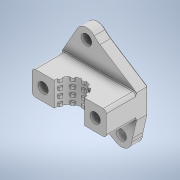
# Autodesk Inventor part: Extruder-Motherboard Cable Harness
Saved by Autodesk Inventor 2020 (Build 240168000, 168)
## iProperties
Created: 2019-12-22
Part Number: Extruder-Motherboard Cable Harness
Material: Generic
Document SubType Name: Modeling
Designer: pepd9
Density: 1 g/cm^3
Appearance: Default
Author: pepd9
Autodesk Inventor part; units mm, degrees
ref_plane "YZ Plane" through (0, 0, 0) normal (1, 0, 0) x (0, 1, 0)
ref_plane "XZ Plane" through (0, 0, 0) normal (0, 1, 0) x (-1, 0, 0)
ref_plane "XY Plane" through (0, 0, 0) normal (0, 0, 1) x (1, 0, 0)
ref_plane "Work Plane1" through (0, 0, 0) normal (0, 0, 1) x (1, 0, 0)
sketch "Sketch1" plane through (0, 0, 0) normal (0, 0, 1) x (1, 0, 0)
  circle A0 centre (228, 110.5) radius 1.1 construction
  circle A1 centre (239.5, 89) radius 1.1 construction
  line L0 (220, 118.5) -> (244.5, 118.5)
  line L1 (244.5, 118.5) -> (244.5, 81)
  line L2 (244.5, 81) -> (220, 81)
  line L3 (220, 81) -> (220, 118.5)
  point P0 (0, 0)
  dimension "d0" = 5
  dimension "d1" = 8
  dimension "d2" = 8
  dimension "d3" = 8
  constraints: 8 end point, 2 parallel, 1 horizontal, 1 perpendicular
  measures "d0" distance from line of A1.centre L1
  measures "d1" distance from line of L3 A0.centre
  measures "d2" distance from line of L2 A1.centre
  measures "d3" distance from line of L0 A0.centre
extrude "Extrusion1" add sketch "Sketch1" along normal blind 3
sketch "Sketch2" plane through (0, 0, 3) normal (0, 0, 1) x (1, 0, 0)
  circle A0 centre (228, 110.5) radius 1.1 projected
  circle A1 centre (239.5, 89) radius 1.1 projected
  point P0 (0, 0)
hole "Hole1" at (228, 110.5, 3) at (239.5, 89, 3) direction (0, 0, -1) diameter 3.4 end through all clearance for "Socket Head Cap Screw" size "M3" standard "Ansi Metric M Profile"
ref_plane "Work Plane2" through (220, 103.5, 0) normal (0, 1, 0) x (1, 0, 0)
sketch "Sketch3" plane through (220, 103.5, 0) normal (0, 1, 0) x (1, 0, 0)
  line L0 (0, -3) -> (24.5, -3) projected
  line L1 (12.25, -3) -> (12.25, -35.3077) construction
  circle A0 centre (12.25, -13) radius 5
  line L2 (24.5, -13) -> (24.5, -3)
  line L3 (7.25, -13) -> (0, -13)
  line L4 (0, -13) -> (0, -3)
  line L5 (0, -13) -> (24.5, -13)
  point P0 (-220, 0)
  point P1 (17.25, -13)
  dimension "d14" = 10
  dimension "d15" = 10
  dimension "d18" = 10
  constraints: 10 end point, 3 vertical, 2 horizontal, 1 horizontal alignment, 1 midpoint, 1 point on line, 3 other
  measures "d15" distance from line of L0 point (12.25, -13)
  measures "d18" distance of L3.end L0.start
extrude "Extrusion2" add sketch "Sketch3" against normal blind 8 contours L0 L2 L5 A0 L3 L4
sketch "Sketch4" plane through (237.25, 103.5, 13) normal (0, 0, 1) x (1, 0, 0)
  line L0 (-17.25, 0) -> (-10, 0) projected
  line L1 (-17.25, 0) -> (-17.25, -8) projected
  line L2 (-10, -8) -> (-17.25, -8) projected
  line L3 (-10, 0) -> (-10, -8) projected
  line L4 (0, 0) -> (7.25, 0) projected
  line L5 (0, 0) -> (0, -8) projected
  line L6 (7.25, -8) -> (0, -8) projected
  line L7 (7.25, 0) -> (7.25, -8) projected
  point P0 (-237.25, -103.5)
  point P1 (-13.625, -4)
  point P2 (3.625, -4)
hole "Hole2" at (223.625, 99.5, 13) at (240.875, 99.5, 13) direction (0, 0, -1) diameter 3.4 end through all clearance for "Socket Head Cap Screw" size "M3" standard "Ansi Metric M Profile"
sketch "Sketch5" plane through (0, 0, 0) normal (0, 0, -1) x (-1, 0, 0)
  circle A0 centre (-240.875, 99.5) radius 1.7 projected
  circle A1 centre (-223.625, 99.5) radius 1.7 projected
  line L0 (-243.625, 101.0877) -> (-240.875, 102.6754)
  line L1 (-240.875, 102.6754) -> (-238.125, 101.0877)
  line L2 (-238.125, 101.0877) -> (-238.125, 97.9123)
  line L3 (-238.125, 97.9123) -> (-240.875, 96.3246)
  line L4 (-240.875, 96.3246) -> (-243.625, 97.9123)
  line L5 (-243.625, 97.9123) -> (-243.625, 101.0877)
  line L6 (-226.375, 101.0877) -> (-223.625, 102.6754)
  line L7 (-223.625, 102.6754) -> (-220.875, 101.0877)
  line L8 (-220.875, 101.0877) -> (-220.875, 97.9123)
  line L9 (-220.875, 97.9123) -> (-223.625, 96.3246)
  line L10 (-223.625, 96.3246) -> (-226.375, 97.9123)
  line L11 (-226.375, 97.9123) -> (-226.375, 101.0877)
  point P0 (0, 0)
  point P1 (-223.625, 99.5)
  dimension "d28" = 5.5
  dimension "d29" = 5.5
  constraints: 24 end point, 2 coincident, 26 other
  measures "d28" distance between parallel lines of L5 L2
  measures "d29" distance between parallel lines of L8 L11
extrude "Extrusion3" cut sketch "Sketch5" against normal blind 5
sketch "Sketch6" plane through (220, 103.5, 0) normal (0, 1, 0) x (1, 0, 0)
  line L0 (0, -3) -> (0, -13) projected
  line L1 (0, -13) -> (7.25, -13) projected
  arc A0 (17.25, -13) -> (7.25, -13) centre (12.25, -13) ccw projected
  line L2 (17.25, -13) -> (24.5, -13) projected
  line L3 (24.5, -13) -> (24.5, -3) projected
  line L4 (0, -3) -> (24.5, -3) projected
  line L5 (7.348, -12.015) -> (7.8461, -11.9714)
  line L6 (7.8461, -11.9714) -> (8.1881, -11.0317)
  line L7 (8.1881, -11.0317) -> (7.8051, -10.7103)
  point P0 (-220, 0)
  dimension "d32" = 5
  dimension "d33" = 45
  dimension "d34" = 115
  dimension "d35" = 1
  dimension "d36" = 0.5
  dimension "d37" = 0.5
  constraints: 6 end point, 2 point on circle
  measures "d32" angle of L5 L1
  measures "d33" angle of L5 L7
  measures "d34" angle of L6 L5
  measures "d35" distance of L5.end L6.end
  measures "d36" distance of L5.start L5.end
  measures "d37" distance of L6.end L7.end
extrude "Extrusion4" add sketch "Sketch6" against normal blind 1 contours A0 L7 L6 L5
pattern_circular "Circular Pattern1" count 5 over 140 about axis through (232.25, 103.5, 13) along (0, -1, 0) of "Extrusion4"
pattern_linear "Rectangular Pattern1" count 4 spacing 2.3 along (0, -1, 0) of "Extrusion4", "Circular Pattern1"
sketch "Sketch7" plane through (0, 0, 3) normal (0, 0, 1) x (1, 0, 0)
  line L0 (220, 103.5) -> (244.5, 103.5) projected
  line L1 (244.5, 103.5) -> (244.5, 118.5) projected
  line L2 (244.5, 118.5) -> (220, 118.5) projected
  line L3 (220, 118.5) -> (220, 103.5) projected
  circle A0 centre (228, 110.5) radius 1.7 projected
  circle A1 centre (239.5, 89) radius 1.7 projected
  line L4 (244.5, 95.5) -> (220, 95.5) projected
  line L5 (220, 95.5) -> (220, 81) projected
  line L6 (220, 81) -> (244.5, 81) projected
  line L7 (244.5, 81) -> (244.5, 95.5) projected
  circle A2 centre (228, 110.5) radius 1.7 projected
  circle A3 centre (228, 110.5) radius 3.5
  circle A4 centre (239.5, 89) radius 3.5
  line L8 (220, 118.5) -> (220, 103.5) projected
  line L9 (244.5, 103.5) -> (231.0594, 112.2)
  line L10 (224.9565, 112.2283) -> (220, 103.5)
  line L11 (244.5, 95.5) -> (220, 95.5) projected
  line L12 (220, 95.5) -> (237.844, 85.9166)
  line L13 (243, 89) -> (244.5, 95.5)
  point P0 (0, 0)
  dimension "d46" = 7
  dimension "d47" = 7
  constraints: 8 end point, 4 point on circle, 2 centre point, 2 coincident, 2 tangent
  measures "d46" diameter of A3
  measures "d47" diameter of A4
extrude "Extrusion5" cut sketch "Sketch7" against normal through all contours L3 L2 L1 L9 A3 L10 | L7 L6 L5 L12 A4 L13
fillet "Fillet1" radius 10 2 edges at (231.0594, 112.2, 1.5) (243, 89, 1.5)
fillet "Fillet2" radius 1 4 edges at (244.5, 103.5, 8) (244.5, 95.5, 8) (220, 95.5, 8) (220, 103.5, 8)
sketch "Sketch8" plane through (0, 0, 5) normal (0, 0, -1) x (-1, 0, 0)
  line L0 (-240.875, 96.3246) -> (-243.625, 97.9123) projected
  line L1 (-238.125, 97.9123) -> (-240.875, 96.3246) projected
  line L2 (-238.125, 101.0877) -> (-238.125, 97.9123) projected
  line L3 (-240.875, 102.6754) -> (-238.125, 101.0877) projected
  line L4 (-243.625, 101.0877) -> (-240.875, 102.6754) projected
  line L5 (-243.625, 97.9123) -> (-243.625, 101.0877) projected
  circle A0 centre (-240.875, 99.5) radius 1.7 projected
  line L6 (-220.875, 97.9123) -> (-223.625, 96.3246) projected
  line L7 (-220.875, 101.0877) -> (-220.875, 97.9123) projected
  line L8 (-223.625, 102.6754) -> (-220.875, 101.0877) projected
  line L9 (-226.375, 101.0877) -> (-223.625, 102.6754) projected
  line L10 (-226.375, 97.9123) -> (-226.375, 101.0877) projected
  line L11 (-223.625, 96.3246) -> (-226.375, 97.9123) projected
  circle A1 centre (-223.625, 99.5) radius 1.7 projected
  line L12 (-235.6121, 101.2) -> (-234.4702, 101.2) projected
  line L13 (-246.7088, 97.8) -> (-235.0412, 97.8)
  line L14 (-235.0412, 97.8) -> (-235.0412, 101.2)
  line L15 (-235.0412, 101.2) -> (-246.7088, 101.2)
  line L16 (-246.7088, 101.2) -> (-246.7088, 97.8)
  line L17 (-246.7088, 97.8) -> (-235.0412, 101.2) construction
  line L18 (-235.0412, 97.8) -> (-246.7088, 101.2) construction
  line L19 (-219.1294, 97.8) -> (-228.1206, 97.8)
  line L20 (-228.1206, 97.8) -> (-228.1206, 101.2)
  line L21 (-228.1206, 101.2) -> (-219.1294, 101.2)
  line L22 (-219.1294, 101.2) -> (-219.1294, 97.8)
  line L23 (-219.1294, 97.8) -> (-228.1206, 101.2) construction
  line L24 (-228.1206, 97.8) -> (-219.1294, 101.2) construction
  line L25 (-237.844, 85.9166) -> (-220, 95.5) projected
  line L26 (-220, 103.5) -> (-220, 95.5) projected
  line L27 (-220, 103.5) -> (-224.9565, 112.2283) projected
  arc A2 (-224.9565, 112.2283) -> (-230.563, 112.8835) centre (-228, 110.5) ccw projected
  arc A3 (-232.4521, 111.2985) -> (-230.563, 112.8835) centre (-237.886, 119.6933) ccw projected
  line L28 (-232.4521, 111.2985) -> (-244.5, 103.5) projected
  line L29 (-244.5, 95.5) -> (-244.5, 103.5) projected
  line L30 (-244.5, 95.5) -> (-243.1723, 89.7464) projected
  arc A4 (-242.9783, 88.6106) -> (-243.1723, 89.7464) centre (-252.9162, 87.4978) ccw projected
  arc A5 (-242.9783, 88.6106) -> (-237.844, 85.9166) centre (-239.5, 89) ccw projected
  line L31 (-220.875, 101.0877) -> (-220.875, 97.9123) projected
  line L32 (-220.875, 97.9123) -> (-223.625, 96.3246) projected
  line L33 (-223.625, 96.3246) -> (-226.375, 97.9123) projected
  line L34 (-226.375, 97.9123) -> (-226.375, 101.0877) projected
  line L35 (-226.375, 101.0877) -> (-223.625, 102.6754) projected
  line L36 (-223.625, 102.6754) -> (-220.875, 101.0877) projected
  line L37 (-238.125, 97.9123) -> (-240.875, 96.3246) projected
  line L38 (-240.875, 96.3246) -> (-243.625, 97.9123) projected
  line L39 (-243.625, 97.9123) -> (-243.625, 101.0877) projected
  line L40 (-243.625, 101.0877) -> (-240.875, 102.6754) projected
  line L41 (-240.875, 102.6754) -> (-238.125, 101.0877) projected
  line L42 (-238.125, 101.0877) -> (-238.125, 97.9123) projected
  circle A6 centre (-228, 110.5) radius 1.7 projected
  circle A7 centre (-239.5, 89) radius 1.7 projected
  point P0 (0, 0)
  point P1 (-223.625, 99.5)
  point P2 (-223.625, 101.2)
  point P3 (-226.1805, 101.2)
  point P4 (-226.1805, 97.8)
  point P5 (-223.625, 97.8)
  point P6 (-221.0695, 101.2)
  point P7 (-221.0695, 97.8)
  point P8 (-238.3195, 101.2)
  point P9 (-240.875, 101.2)
  point P10 (-240.875, 97.8)
  point P11 (-238.3195, 97.8)
  point P12 (-243.4305, 101.2)
  point P13 (-243.4305, 97.8)
  dimension "d52" = 3.4
  dimension "d53" = 3.4
  constraints: 24 end point, 5 midpoint, 4 parallel, 2 horizontal, 2 perpendicular
  measures "d52" distance of L14.end L13.end
  measures "d53" distance of L19.end L20.end
extrude "Extrusion6" cut sketch "Sketch8" against normal blind 0.5 contours L0 L5 L4 L15 A0 L13 | L13 A0 L15 L3 L2 L1 | L19 A1 L21 L8 L7 L6 | L19 L11 L10 L9 L21 A1
sketch "Sketch9" plane through (0, 0, 5.5) normal (0, 0, -1) x (-1, 0, 0)
  line L0 (-240.875, 101.2) -> (-238.3195, 101.2) projected
  arc A0 (-240.875, 97.8) -> (-240.875, 101.2) centre (-240.875, 99.5) ccw projected
  line L1 (-238.3195, 97.8) -> (-240.875, 97.8) projected
  line L2 (-238.125, 97.9123) -> (-238.3195, 97.8) projected
  line L3 (-238.125, 101.0877) -> (-238.125, 97.9123) projected
  line L4 (-238.3195, 101.2) -> (-238.125, 101.0877) projected
  line L5 (-243.4305, 101.2) -> (-240.875, 101.2) projected
  line L6 (-243.625, 101.0877) -> (-243.4305, 101.2) projected
  line L7 (-243.625, 97.9123) -> (-243.625, 101.0877) projected
  line L8 (-243.4305, 97.8) -> (-243.625, 97.9123) projected
  line L9 (-240.875, 97.8) -> (-243.4305, 97.8) projected
  arc A1 (-240.875, 101.2) -> (-240.875, 97.8) centre (-240.875, 99.5) ccw projected
  line L10 (-226.1805, 101.2) -> (-223.625, 101.2) projected
  line L11 (-226.375, 101.0877) -> (-226.1805, 101.2) projected
  line L12 (-226.375, 97.9123) -> (-226.375, 101.0877) projected
  line L13 (-226.1805, 97.8) -> (-226.375, 97.9123) projected
  line L14 (-223.625, 97.8) -> (-226.1805, 97.8) projected
  arc A2 (-223.625, 101.2) -> (-223.625, 97.8) centre (-223.625, 99.5) ccw projected
  line L15 (-221.0695, 101.2) -> (-220.875, 101.0877) projected
  line L16 (-223.625, 101.2) -> (-221.0695, 101.2) projected
  arc A3 (-223.625, 97.8) -> (-223.625, 101.2) centre (-223.625, 99.5) ccw projected
  line L17 (-221.0695, 97.8) -> (-223.625, 97.8) projected
  line L18 (-220.875, 97.9123) -> (-221.0695, 97.8) projected
  line L19 (-220.875, 101.0877) -> (-220.875, 97.9123) projected
  line L20 (-239.175, 101.2) -> (-242.575, 101.2)
  line L21 (-242.575, 101.2) -> (-242.575, 97.8)
  line L22 (-242.575, 97.8) -> (-239.175, 97.8)
  line L23 (-239.175, 97.8) -> (-239.175, 101.2)
  line L24 (-239.175, 101.2) -> (-242.575, 97.8) construction
  line L25 (-242.575, 101.2) -> (-239.175, 97.8) construction
  line L26 (-225.325, 101.2) -> (-221.925, 101.2)
  line L27 (-221.925, 101.2) -> (-221.925, 97.8)
  line L28 (-221.925, 97.8) -> (-225.325, 97.8)
  line L29 (-225.325, 97.8) -> (-225.325, 101.2)
  line L30 (-225.325, 101.2) -> (-221.925, 97.8) construction
  line L31 (-221.925, 101.2) -> (-225.325, 97.8) construction
  point P0 (0, 0)
  dimension "d56" = 3.4
  dimension "d57" = 3.4
  dimension "d58" = 3.4
  dimension "d59" = 3.4
  constraints: 24 end point, 4 midpoint, 4 parallel, 2 horizontal, 2 perpendicular
  measures "d56" distance of L22.end L21.end
  measures "d57" distance of L21.end L20.end
  measures "d58" distance of L27.end L28.end
  measures "d59" distance of L26.end L27.end
extrude "Extrusion7" cut sketch "Sketch9" against normal blind 0.5 contours L0 L23 A0 | A1 L21 L5 | A0 A1 | L23 L1 A0 | A1 L9 L21 | L10 A2 L29 | A3 A2 | L16 L27 A3 | A2 L14 L29 | L27 L17 A3
move faces "Move1" translate (0, 0, -0.75) faces at (234.2003, 95.2634, 0)
chamfer "Chamfer1" distance 0.25 angle 45 22 edges at (238.476, 107.3993, -0.75) (231.4585, 112.0326, -0.75) (227.5938, 113.9763, -0.75) (222.4782, 107.8642, -0.75) (244.5, 99.5, -0.75) (243.8361, 92.6232, -0.75) (243.0589, 89.1813, -0.75) (241.1262, 85.9007, -0.75) (228.922, 90.7083, -0.75) (242.25, 97.1184, -0.75) (239.5, 97.1184, -0.75) (238.125, 99.5, -0.75) (239.5, 101.8816, -0.75) (242.25, 101.8816, -0.75) (243.625, 99.5, -0.75) (226.375, 99.5, -0.75) (225, 101.8816, -0.75) (222.25, 101.8816, -0.75) (220.875, 99.5, -0.75) (222.25, 97.1184, -0.75) (220, 99.5, -0.75) (225, 97.1184, -0.75)
chamfer "Chamfer2" distance 0.25 angle 45 6 edges at (232.25, 95.5, 3) (220.2929, 95.7929, 3) (244.2071, 95.7929, 3) (232.25, 103.5, 3) (244.2071, 103.2071, 3) (220.2929, 103.2071, 3)
body "Solid1"
